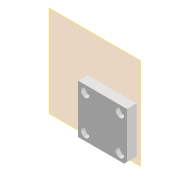
# Autodesk Inventor part: 30_cellSTORM_UC2_Chip_holder_base
Saved by Autodesk Inventor 2022 (Build 260153000, 153)
## iProperties
Created: 2021-11-19
Part Number: 30_cellSTORM_UC2_Chip_holder_base
Material: Generic
Document SubType Name: Modeling
Designer: diederichbenedict
Density: 1 g/cm^3
Appearance: Default
Author: diederichbenedict
Autodesk Inventor part; units mm, degrees
ref_plane "YZ Plane" through (0, 0, 0) normal (1, 0, 0) x (0, 1, 0)
ref_plane "XZ Plane" through (0, 0, 0) normal (0, 1, 0) x (-1, 0, 0)
ref_plane "XY Plane" through (0, 0, 0) normal (0, 0, 1) x (1, 0, 0)
ref_plane "Work Plane1" through (0, 0, 0) normal (0, 0, 1) x (1, 0, 0)
sketch "Sketch1" plane through (0, 0, 0) normal (0, 0, 1) x (1, 0, 0)
  circle A0 centre (25, -10) radius 1.45 projected
  circle A1 centre (-25, -10) radius 1.45 projected
  circle A2 centre (-25, 10) radius 1.45 projected
  circle A3 centre (25, 10) radius 1.45 projected
  circle A4 centre (-10, -25) radius 1.45 projected
  circle A5 centre (-10, 25) radius 1.45 projected
  circle A6 centre (10, 25) radius 1.45 projected
  circle A7 centre (10, -25) radius 1.45 projected
  circle A8 centre (-25, 25) radius 2.325 projected
  circle A9 centre (25, -25) radius 2.325 projected
  circle A10 centre (-25, -25) radius 2.325 projected
  circle A11 centre (25, 25) radius 2.325 projected
  line L0 (28, 30) -> (30, 28) projected
  line L1 (28, 30) -> (-28, 30) projected
  line L2 (-30, 28) -> (-28, 30) projected
  line L3 (-30, 28) -> (-30, -28) projected
  line L4 (-28, -30) -> (-30, -28) projected
  line L5 (-28, -30) -> (28, -30) projected
  line L6 (30, -28) -> (28, -30) projected
  line L7 (30, -28) -> (30, 28) projected
  circle A12 centre (-17.5, -17.5) radius 1.95 projected
  circle A13 centre (17.5, 17.5) radius 1.95 projected
  circle A14 centre (17.5, -17.5) radius 1.95 projected
  circle A15 centre (-17.5, 17.5) radius 1.95 projected
  circle A16 centre (0, 0) radius 7.5 projected
  line L8 (30, -30) -> (-5, -30)
  line L9 (-5, -30) -> (-5, 5)
  line L10 (-5, 5) -> (30, 5)
  line L11 (30, 5) -> (30, -30)
  point P0 (0, 0)
  dimension "d0" = 35
  dimension "d1" = 35
  constraints: 8 end point, 2 parallel, 1 horizontal, 1 perpendicular, 1 point on line
  measures "d0" distance of L9.end L10.end
  measures "d1" distance of L8.end L9.end
extrude "Extrusion1" add sketch "Sketch1" along normal blind 7 contours A0 | A7 | A9 | L7 L6 L5 L9 A16 L10 | A16 L9 L10 | A14 picked at (1.7753, -1.9143)
sketch "Sketch2" plane through (0, 0, 7) normal (0, 0, 1) x (1, 0, 0)
  line L0 (9.7965, -11.8691) -> (15.0465, -11.8691) projected
  line L1 (-5, 5) -> (-5, -30) projected
  line L2 (-5, -30) -> (28, -30) projected
  line L3 (28, -30) -> (30, -28) projected
  line L4 (30, -28) -> (30, 5) projected
  line L5 (30, 5) -> (-5, 5) projected
  circle A0 centre (12.5, -12.5) radius 17.5
  line L6 (25, -25) -> (0, -25)
  line L7 (0, -25) -> (0, 0)
  line L8 (0, 0) -> (25, 0)
  line L9 (25, 0) -> (25, -25)
  line L10 (25, -25) -> (0, 0) construction
  line L11 (0, -25) -> (25, 0) construction
  dimension "d4" = 25
  dimension "d5" = 25
  constraints: 12 end point, 3 tangent, 2 midpoint, 2 parallel, 1 centre point, 1 horizontal, 1 perpendicular
  measures "d4" distance of L7.end L8.end
  measures "d5" distance of L6.end L7.end
hole "Hole1" at (25, 0, 7) at (0, -25, 7) at (0, 0, 7) at (25, -25, 7) direction (0, 0, -1) diameter 3 end through all counterbore diameter 6 counterbore depth 3
sketch "Sketch3" plane through (0, 0, 7) normal (0, 0, 1) x (1, 0, 0)
  circle A0 centre (18.5383, 7.9631) radius 1.4 construction
  circle A1 centre (8.5565, 1.2345) radius 2.95 construction
  circle A2 centre (8.5565, -23.0142) radius 2.95 construction
  circle A3 centre (29.5565, -10.8899) radius 2.95 construction
  line L0 (4.5565, -28.3465) -> (33.5565, -28.3465) construction
  line L1 (4.5565, 11.2345) -> (4.5565, -28.3465) construction
  line L2 (33.5565, 11.2345) -> (4.5565, 11.2345) construction
  line L3 (33.5565, -28.3465) -> (33.5565, 11.2345) construction
  line L4 (-5, 5) -> (-5, -30) construction
  line L5 (30, 5) -> (-5, 5) construction
  line L6 (30, -28) -> (30, 5) construction
  circle A4 centre (12.5, -12.5) radius 17.5 construction
  line L7 (26.5, -12.5) -> (5.5, -24.6244) construction
  line L8 (5.5, -24.6244) -> (5.5, -0.3756) construction
  line L9 (5.5, -0.3756) -> (26.5, -12.5) construction
  point P0 (0, 0)
  dimension "d13" = 12.1244
  dimension "d14" = 21
  dimension "d15" = 21
  constraints: 6 end point, 3 tangent, 1 centre point, 1 coincident, 1 parallel, 7 other
  measures "d13" vertical distance of A1.centre A3.centre
  measures "d14" horizontal distance of A1.centre A3.centre
  measures "d15" distance from line of L8 L7.start
hole "Hole2" at (26.5, -12.5, 7) at (5.5, -24.6244, 7) at (5.5, -0.3756, 7) direction (0, 0, -1) diameter 2.8 end through all
body "Solid1"
